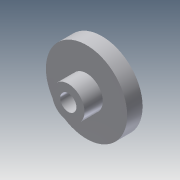
# Autodesk Inventor part: otaceni_packy_microservo
Saved by Autodesk Inventor 2013 (Build 170138000, 138)
## iProperties
Created: 2013-02-02
Part Number: otaceni_packy_microservo
Material: Generic
Document SubType Name: Modeling
Designer: idle-rug
Density: 1 g/cm^3
Author: idle-rug
Autodesk Inventor part; units mm, degrees
ref_plane "YZ Plane" through (0, 0, 0) normal (1, 0, 0) x (0, 1, 0)
ref_plane "XZ Plane" through (0, 0, 0) normal (0, 1, 0) x (-1, 0, 0)
ref_plane "XY Plane" through (0, 0, 0) normal (0, 0, 1) x (1, 0, 0)
sketch "Sketch1" plane through (0, 0, 0) normal (0, 1, 0) x (-1, 0, 0)
  circle A0 centre (0, 0) radius 10
  dimension "d0" = 20
  constraints: 1 centre point, 1 coincident
  measures "d0" diameter of A0
extrude "Extrusion1" add sketch "Sketch1" along normal blind 1.8
sketch "Sketch3" plane through (0, 1.8, 0) normal (0, 1, 0) x (1, 0, 0)
  circle A0 centre (0, 0) radius 10 projected
  circle A1 centre (0, 0) radius 3.5
  circle A2 centre (0, 0) radius 2.5
  dimension "d3" = 7
  dimension "d4" = 5
  constraints: 2 centre point, 2 coincident
  measures "d3" diameter of A1
  measures "d4" diameter of A2
extrude "Extrusion2" add sketch "Sketch3" along normal blind 2.4 contours A1
sketch "Sketch4" plane through (0, 0, 0) normal (0, -1, 0) x (1, 0, 0)
  circle A0 centre (0, 0) radius 10 projected
  line L0 (0, 0) -> (6.3, 0)
  circle A1 centre (6.3, 0) radius 1.5
  dimension "d7" = 6.3
  dimension "d8" = 3
  constraints: 2 end point, 1 centre point, 1 coincident, 1 horizontal
  measures "d7" distance of L0.start L0.end
  measures "d8" diameter of A1
extrude "Extrusion3" cut sketch "Sketch4" against normal blind 2.4 contours A1
sketch "Sketch5" plane through (0, 0, 0) normal (0, -1, 0) x (1, 0, 0)
  circle A0 centre (0, 0) radius 10 projected
  line L0 (0, 0) -> (-6.3, 0)
  circle A1 centre (-6.3, 0) radius 1.5
  dimension "d11" = 6.3
  dimension "d12" = 3
  constraints: 2 end point, 1 centre point, 1 coincident, 1 horizontal
  measures "d11" distance of L0.start L0.end
  measures "d12" diameter of A1
extrude "Extrusion4" cut sketch "Sketch5" against normal blind 2 contours A1
sketch "Sketch6" plane through (0, 0, 0) normal (0, -1, 0) x (1, 0, 0)
  circle A0 centre (-6.3, 0) radius 1.5 projected
  circle A1 centre (6.3, 0) radius 1.5 projected
extrude "Extrusion5" add sketch "Sketch6" against normal blind 1.8
sketch "Sketch7" plane through (0, 0, 0) normal (0, -1, 0) x (1, 0, 0)
  circle A0 centre (0, 0) radius 10 projected
extrude "Extrusion6" add sketch "Sketch7" along normal blind 2
sketch "Sketch8" plane through (0, -2, 0) normal (0, -1, 0) x (1, 0, 0)
  circle A0 centre (0, 0) radius 10 projected
  circle A1 centre (0, 0) radius 4
  circle A2 centre (0, 0) radius 2
  dimension "d19" = 8
  dimension "d20" = 4
  constraints: 2 centre point, 2 coincident
  measures "d19" diameter of A1
  measures "d20" diameter of A2
extrude "Extrusion7" add sketch "Sketch8" along normal blind 4.5 contours A1
body "Solid1"
